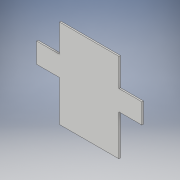
# Autodesk Inventor part: 20Gen2PlatePart
Saved by Autodesk Inventor 2019 (Build 230136000, 136)
## iProperties
Created: 2017-12-06
Part Number: 20Gen2PlatePart
Material: Generic
Document SubType Name: Modeling
Designer: User
Density: 1 g/cm^3
Appearance: Default
Mass: 688.034 g
Surface Area: 2294.14 cm^2
Volume: 688.034 cm^3
Author: User
Autodesk Inventor part; units mm, degrees
ref_plane "YZ Plane" through (0, 0, 0) normal (1, 0, 0) x (0, 1, 0)
ref_plane "Work Plane32" through (254, 330.2, 0) normal (0, 0, -1) x (-1, 0, 0)
sketch "Sketch36" plane through (254, 330.2, 0) normal (0, 0, -1) x (-1, 0, 0)
  line L0 (254, -363.855) -> (254, -196.85) projected
  line L1 (0, 0) -> (0, -114.3) projected
  line L2 (254, -363.855) -> (0, -363.855)
  line L3 (0, -363.855) -> (0, 0)
  line L4 (0, 0) -> (254, 0)
  line L5 (254, 0) -> (254, -363.855)
  line L6 (342.9, -196.85) -> (342.9, -114.3) projected
  line L7 (342.9, -196.85) -> (254, -196.85)
  line L8 (254, -196.85) -> (254, -114.3)
  line L9 (254, -114.3) -> (342.9, -114.3)
  line L10 (342.9, -114.3) -> (342.9, -196.85)
  line L11 (-31.75, -363.855) -> (254, -363.855) projected
  line L12 (0, -314.325) -> (0, -196.85) projected
  line L13 (-31.75, -363.855) -> (0, -363.855)
  line L14 (0, -363.855) -> (0, -314.325)
  line L15 (0, -314.325) -> (-31.75, -314.325)
  line L16 (-31.75, -314.325) -> (-31.75, -363.855)
  line L17 (0, -196.85) -> (-88.9, -196.85)
  line L18 (-88.9, -196.85) -> (-88.9, -114.3)
  line L19 (-88.9, -114.3) -> (0, -114.3)
  line L20 (0, -114.3) -> (0, -196.85)
  dimension "d412" = 82.55
  dimension "d413" = 254
  dimension "d414" = 31.75
  constraints: 32 end point, 8 parallel, 4 horizontal, 4 perpendicular, 1 point on line
  measures "d412" distance between parallel lines of L9 L7
  measures "d413" distance between parallel lines of L5 L1
  measures "d414" distance between parallel lines of L3 L16
extrude "Extrusion20" add sketch "Sketch36" along normal blind 6.35
ref_plane "Work Plane28" through (254, 330.2, -6.35) normal (0, 0, -1) x (-1, 0, 0)
sketch "Sketch39" plane through (254, 330.2, -6.35) normal (0, 0, -1) x (-1, 0, 0)
  line L0 (0, -196.85) -> (0, -314.325) projected
  line L1 (0, -196.85) -> (5.08, -196.85)
  line L2 (5.08, -196.85) -> (5.08, -314.325)
  line L3 (5.08, -314.325) -> (0, -314.325)
  line L4 (0, -314.325) -> (0, -196.85)
  line L5 (254, -363.855) -> (254, -196.85) projected
  line L6 (-31.75, -363.855) -> (254, -363.855) projected
  line L7 (254, -196.85) -> (248.92, -196.85)
  line L8 (248.92, -196.85) -> (248.92, -363.855)
  line L9 (248.92, -363.855) -> (254, -363.855)
  line L10 (254, -363.855) -> (254, -196.85)
  line L11 (0, -114.3) -> (-88.9, -114.3) projected
  line L12 (254, 0) -> (0, 0) projected
  line L13 (0, -114.3) -> (5.08, -114.3)
  line L14 (5.08, -114.3) -> (5.08, 0)
  line L15 (5.08, 0) -> (0, 0)
  line L16 (0, 0) -> (0, -114.3)
  line L17 (254, 0) -> (248.92, 0)
  line L18 (248.92, 0) -> (248.92, -114.3)
  line L19 (248.92, -114.3) -> (254, -114.3)
  line L20 (254, -114.3) -> (254, 0)
  point P0 (254, -330.2)
  dimension "d415" = 5.08
  dimension "d416" = 5.08
  dimension "d417" = 5.08
  constraints: 32 end point, 8 parallel, 4 horizontal, 4 perpendicular, 4 point on line
  measures "d415" distance of L2.end L3.end
  measures "d416" distance of L9.end L8.end
  measures "d417" distance of L15.end L14.end
extrude "Extrusion22" cut sketch "Sketch39" against normal blind 6.35
sketch "Sketch41" plane through (254, 330.2, 0) normal (0, 0, 1) x (1, 0, 0)
  line L0 (-5.08, -314.325) -> (31.75, -314.325) projected
  line L1 (31.75, -363.855) -> (-248.92, -363.855) projected
  line L2 (31.75, -314.325) -> (-5.08, -314.325)
  line L3 (-5.08, -314.325) -> (-5.08, -363.855)
  line L4 (-5.08, -363.855) -> (31.75, -363.855)
  line L5 (31.75, -363.855) -> (31.75, -314.325)
  point P0 (-254, -330.2)
  dimension "d448" = 36.83
  constraints: 8 end point, 2 parallel, 1 horizontal, 1 perpendicular, 1 point on line
  measures "d448" distance of L4.end L3.end
extrude "Extrusion24" cut sketch "Sketch41" against normal blind 6.35
body "Solid1"
